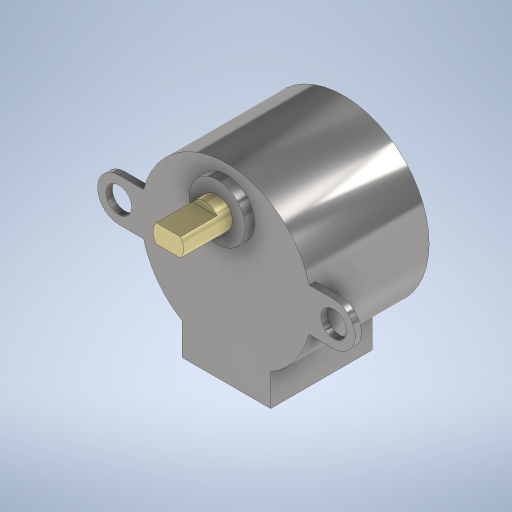
# Autodesk Inventor part: 스텝모터
Saved by Autodesk Inventor 2023.1 (Build 271208000, 208)
## iProperties
Created: 2022-08-14
Part Number: 스텝모터
Material: 일반
Document SubType Name: Modeling
Designer: fly01
Density: 1 g/cm^3
Appearance: 기본값
Author: fly01
Autodesk Inventor part; units mm, degrees
ref_plane "YZ Plane" through (0, 0, 0) normal (1, 0, 0) x (0, 1, 0)
ref_plane "XZ Plane" through (0, 0, 0) normal (0, 1, 0) x (-1, 0, 0)
ref_plane "XY Plane" through (0, 0, 0) normal (0, 0, 1) x (1, 0, 0)
sketch "스케치1" plane through (0, 0, 0) normal (0, 0, 1) x (1, 0, 0)
  circle A0 centre (0, 0) radius 14
  line L0 (-7.25, -10.8235) -> (7.25, -10.8235) construction
  line L1 (7.25, -10.8235) -> (7.25, -17.1765)
  line L2 (7.25, -17.1765) -> (-7.25, -17.1765)
  line L3 (-7.25, -17.1765) -> (-7.25, -10.8235)
  line L4 (-7.25, -10.8235) -> (7.25, -17.1765) construction
  line L5 (7.25, -10.8235) -> (-7.25, -17.1765) construction
  line L6 (7.25, -11.9765) -> (7.25, -17.1765)
  line L7 (0, -14) -> (0, 0)
  point P0 (-7.25, -11.9765)
  dimension "d0" = 28
  dimension "d1" = 5.2
  dimension "d2" = 14.5
  constraints: 16 end point, 2 midpoint, 2 parallel, 2 point on circle, 1 centre point, 1 coincident, 1 collinear, 1 horizontal, 1 perpendicular, 1 point on line, 1 vertical
  measures "d0" diameter of A0
  measures "d1" distance of L1.end L6.start
  measures "d2" distance of L1.end L2.end
extrude "돌출1" add sketch "스케치1" against normal blind 19.2 contours A0
extrude "돌출2" add sketch "스케치1" against normal blind 16.6 contours A0 L1 L2 L3
sketch "스케치2" plane through (0, 0, 0) normal (0, 0, 1) x (1, 0, 0)
  circle A0 centre (-17.6, 0) radius 2.1
  circle A1 centre (-17.6, 0) radius 3.5
  line L0 (-17.6, 3.5) -> (-13.5554, 3.5)
  line L1 (-17.6, -3.5) -> (-13.5554, -3.5)
  line L2 (-17.6, 0) -> (0, 0)
  arc A2 (7.25, -11.9765) -> (-7.25, -11.9765) centre (0, 0) ccw projected
  dimension "d7" = 4.2
  dimension "d8" = 7
  dimension "d9" = 17.6
  constraints: 6 end point, 4 point on circle, 3 horizontal, 2 centre point, 2 tangent, 1 coincident
  measures "d7" diameter of A0
  measures "d8" diameter of A1
  measures "d9" distance of L2.start L2.end
extrude "돌출3" add sketch "스케치2" against normal blind 1
mirror "미러1" about plane through (0, 0, 0) normal (1, 0, 0) of "돌출3"
sketch "스케치3" plane through (0, 0, 0) normal (0, 0, 1) x (1, 0, 0)
  circle A0 centre (0, 7.8) radius 4.6
  line L0 (0, 12.4) -> (0, 14)
  arc A1 (13.5554, 3.5) -> (-13.5554, 3.5) centre (0, 0) ccw projected
  line L1 (0, 7.8) -> (0, 0)
  point P0 (0, 14)
  dimension "d12" = 9.2
  dimension "d13" = 1.6
  constraints: 4 end point, 3 vertical alignment, 2 point on circle, 2 vertical, 2 other
  measures "d13" distance of L0.start L0.end
extrude "돌출4" add sketch "스케치3" along normal blind 1.5
sketch "스케치4" plane through (0, 7.8, 1.5) normal (0, 0, 1) x (1, 0, 0)
  circle A0 centre (0, 0) radius 4.6 projected
  circle A1 centre (0, 0) radius 2.5
  point P0 (0, -7.8)
  dimension "d16" = 5
  constraints: 1 centre point, 1 coincident
  measures "d16" diameter of A1
extrude "돌출5" add sketch "스케치4" along normal blind 8 contours A1
sketch "스케치5" plane through (0, 7.8, 9.5) normal (0, 0, 1) x (1, 0, 0)
  circle A0 centre (0, 0) radius 2.5 projected
  line L0 (-2.5, 1.5) -> (2.5, 1.5)
  line L1 (2.5, 1.5) -> (2.5, -1.5)
  line L2 (2.5, -1.5) -> (-2.5, -1.5)
  line L3 (-2.5, -1.5) -> (-2.5, 1.5)
  line L4 (-2.5, 1.5) -> (2.5, -1.5) construction
  line L5 (2.5, 1.5) -> (-2.5, -1.5) construction
  point P0 (0, -7.8)
  point P1 (2, -1.5)
  point P2 (-2, -1.5)
  point P3 (-2, 1.5)
  point P4 (2, 1.5)
  dimension "d19" = 3
  constraints: 12 end point, 2 midpoint, 2 parallel, 1 horizontal, 1 perpendicular
  measures "d19" distance of L0.end L1.end
extrude "돌출6" cut sketch "스케치5" against normal blind 6 contours L0 A0 | A0 L2
ref_plane "작업 평면1" through (0, 0, 0) normal (1, 0, 0) x (0, 1, 0)
